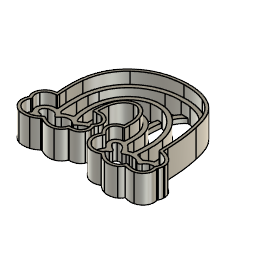
Rainbow v8 (Autodesk Fusion 360 design; units mm, degrees)
Autodesk Fusion 360 part; units mm, degrees
note: some values were not read from the file. Set by a fixed rule: which sketch regions a step uses.
(part 1 of 4)
sketch "Sketch1" plane through (0, 0, 0) normal (0, 0, 1) x (1, 0, 0)
  spline S0 degree 3 poles (40.6021, -45.3763) (39.7141, -45.1374) (38.685, -44.5376) (37.8366, -43.7642) knots 0 0 0 0 1 1 1 1
  line L0 (37.8366, -43.7642) -> (37.0528, -43.0498)
  line L1 (37.0528, -43.0498) -> (36.4497, -43.413)
  spline S1 degree 3 poles (36.4497, -43.413) (34.0687, -44.8468) (31.3596, -44.1594) (29.9199, -41.7563) knots 0 0 0 0 1 1 1 1
  spline S2 degree 3 poles (29.9199, -41.7563) (29.1248, -40.4292) (29.1935, -38.9614) (30.1335, -37.1915) knots 0 0 0 0 1 1 1 1
  line L2 (30.1335, -37.1915) -> (30.6349, -36.2474)
  line L3 (30.6349, -36.2474) -> (29.844, -35.4477)
  spline S3 degree 3 poles (29.844, -35.4477) (28.95, -34.5436) (28.6612, -33.9245) (28.6688, -32.9285) knots 0 0 0 0 1 1 1 1
  spline S4 degree 3 poles (28.6688, -32.9285) (28.6799, -31.4768) (29.8956, -30.2337) (31.6248, -29.9058) knots 0 0 0 0 1 1 1 1
  spline S5 degree 3 poles (31.6248, -29.9058) (31.9315, -29.8476) (32.2095, -29.7731) (32.2426, -29.7402) knots 0 0 0 0 1 1 1 1
  spline S6 degree 3 poles (32.2426, -29.7402) (32.2756, -29.7073) (32.3172, -28.7609) (32.3351, -27.6372) knots 0 0 0 0 1 1 1 1
  spline S7 degree 3 poles (32.3351, -27.6372) (32.3724, -25.2889) (32.226, -24.0781) (31.7223, -22.5668) knots 0 0 0 0 1 1 1 1
  spline S8 degree 3 poles (31.7223, -22.5668) (31.0329, -20.4985) (29.7724, -18.9275) (28.1619, -18.1295) knots 0 0 0 0 1 1 1 1
  spline S9 degree 3 poles (28.1619, -18.1295) (26.9869, -17.5472) (26.1291, -17.4128) (25.0253, -17.6379) knots 0 0 0 0 1 1 1 1
  spline S10 degree 3 poles (25.0253, -17.6379) (22.1239, -18.2295) (19.9977, -20.7694) (19.2274, -24.5637) knots 0 0 0 0 1 1 1 1
  spline S11 degree 3 poles (19.2274, -24.5637) (18.8969, -26.1921) (18.6739, -29.7666) (18.8842, -30.0674) knots 0 0 0 0 1 1 1 1
  spline S12 degree 3 poles (18.8842, -30.0674) (18.9324, -30.1364) (19.5594, -30.1752) (20.5764, -30.1721) knots 0 0 0 0 1 1 1 1
  spline S13 degree 3 poles (20.5764, -30.1721) (22.0397, -30.1678) (22.246, -30.1902) (22.7653, -30.4097) knots 0 0 0 0 1 1 1 1
  spline S14 degree 3 poles (22.7653, -30.4097) (24.0541, -30.9546) (24.7351, -31.7681) (24.8235, -32.8684) knots 0 0 0 0 1 1 1 1
  spline S15 degree 3 poles (24.8235, -32.8684) (24.8681, -33.424) (24.8348, -33.6203) (24.6146, -34.1013) knots 0 0 0 0 1 1 1 1
  spline S16 degree 3 poles (24.6146, -34.1013) (24.4706, -34.4159) (24.1763, -34.8686) (23.9606, -35.1073) knots 0 0 0 0 1 1 1 1
  line L4 (23.9606, -35.1073) -> (23.5686, -35.5413)
  line L5 (23.5686, -35.5413) -> (23.8705, -36.1371)
  spline S17 degree 3 poles (23.8705, -36.1371) (24.1088, -36.6075) (24.1803, -36.9044) (24.2098, -37.5469) knots 0 0 0 0 1 1 1 1
  spline S18 degree 3 poles (24.2098, -37.5469) (24.2439, -38.2891) (24.2182, -38.4195) (23.9188, -39.0278) knots 0 0 0 0 1 1 1 1
  spline S19 degree 3 poles (23.9188, -39.0278) (23.2828, -40.3197) (22.3235, -40.8384) (20.4042, -40.9282) knots 0 0 0 0 1 1 1 1
  line L6 (20.4042, -40.9282) -> (19.2417, -40.9826)
  line L7 (19.2417, -40.9826) -> (19.1816, -41.2833)
  spline S20 degree 3 poles (19.1816, -41.2833) (18.9486, -42.4484) (17.823, -43.6952) (16.6466, -44.0912) knots 0 0 0 0 1 1 1 1
  spline S21 degree 3 poles (16.6466, -44.0912) (15.1238, -44.6038) (13.5396, -44.3544) (11.5251, -43.2849) knots 0 0 0 0 1 1 1 1
  spline S22 degree 3 poles (11.5251, -43.2849) (10.3126, -42.6412) (10.4824, -42.625) (9.5048, -43.4776) knots 0 0 0 0 1 1 1 1
  spline S23 degree 3 poles (9.5048, -43.4776) (8.7123, -44.1689) (7.8391, -44.6696) (6.8696, -44.9888) knots 0 0 0 0 1 1 1 1
  spline S24 degree 3 poles (6.8696, -44.9888) (5.7759, -45.3488) (3.9668, -45.3933) (3.0651, -45.0822) knots 0 0 0 0 1 1 1 1
  spline S25 degree 3 poles (3.0651, -45.0822) (0.3591, -44.1486) (-0.7772, -41.3233) (0.6383, -39.0481) knots 0 0 0 0 1 1 1 1
  line L8 (0.6383, -39.0481) -> (0.884, -38.6532)
  line L9 (0.884, -38.6532) -> (0.5251, -38.0579)
  spline S26 degree 3 poles (0.5251, -38.0579) (-0.1869, -36.8769) (-0.2404, -35.9922) (0.3271, -34.7796) knots 0 0 0 0 1 1 1 1
  spline S27 degree 3 poles (0.3271, -34.7796) (1.1017, -33.1242) (2.7938, -32.1034) (4.7746, -32.0964) knots 0 0 0 0 1 1 1 1
  line L10 (4.7746, -32.0964) -> (5.2854, -32.0946)
  line L11 (5.2854, -32.0946) -> (5.222, -31.0262)
  spline S28 degree 3 poles (5.222, -31.0262) (5.1871, -30.4386) (5.1039, -29.1135) (5.0371, -28.0816) knots 0 0 0 0 1 1 1 1
  spline S29 degree 3 poles (5.0371, -28.0816) (4.8966, -25.9098) (4.9658, -22.8542) (5.1997, -20.8963) knots 0 0 0 0 1 1 1 1
  spline S30 degree 3 poles (5.1997, -20.8963) (5.8689, -15.2961) (8.1545, -10.5999) (11.9514, -7.0234) knots 0 0 0 0 1 1 1 1
  spline S31 degree 3 poles (11.9514, -7.0234) (16.4317, -2.8033) (22.1029, -0.554) (28.8108, -0.3366) knots 0 0 0 0 1 1 1 1
  spline S32 degree 3 poles (28.8108, -0.3366) (32.5622, -0.2151) (35.8702, -0.8038) (38.5701, -2.0736) knots 0 0 0 0 1 1 1 1
  spline S33 degree 3 poles (38.5701, -2.0736) (39.9873, -2.7401) (40.9328, -3.3672) (41.9013, -4.2831) knots 0 0 0 0 1 1 1 1
  spline S34 degree 3 poles (41.9013, -4.2831) (44.1778, -6.4358) (45.3916, -9.0372) (46.5245, -14.1912) knots 0 0 0 0 1 1 1 1
  spline S35 degree 3 poles (46.5245, -14.1912) (47.5435, -18.8273) (47.9159, -21.9078) (48.1971, -28.0295) knots 0 0 0 0 1 1 1 1
  spline S36 degree 3 poles (48.1971, -28.0295) (48.259, -29.3767) (48.3316, -30.5812) (48.3583, -30.7061) knots 0 0 0 0 1 1 1 1
  spline S37 degree 3 poles (48.3583, -30.7061) (48.3975, -30.889) (48.524, -30.9562) (49.0062, -31.0504) knots 0 0 0 0 1 1 1 1
  spline S38 degree 3 poles (49.0062, -31.0504) (51.4412, -31.526) (53.0985, -32.5346) (53.8053, -33.9708) knots 0 0 0 0 1 1 1 1
  spline S39 degree 3 poles (53.8053, -33.9708) (54.0458, -34.4594) (54.0871, -34.6749) (54.0852, -35.4301) knots 0 0 0 0 1 1 1 1
  spline S40 degree 3 poles (54.0852, -35.4301) (54.0832, -36.197) (54.0369, -36.4233) (53.7407, -37.1142) knots 0 0 0 0 1 1 1 1
  line L12 (53.7407, -37.1142) -> (53.3985, -37.9124)
  line L13 (53.3985, -37.9124) -> (53.5734, -38.5139)
  spline S41 degree 3 poles (53.5734, -38.5139) (54.1518, -40.5038) (52.8727, -42.5116) (50.6477, -43.1059) knots 0 0 0 0 1 1 1 1
  spline S42 degree 3 poles (50.6477, -43.1059) (49.6551, -43.3711) (48.4974, -43.2512) (46.8656, -42.7141) knots 0 0 0 0 1 1 1 1
  spline S43 degree 3 poles (46.8656, -42.7141) (46.1378, -42.4746) (45.9769, -42.523) (45.8572, -43.0173) knots 0 0 0 0 1 1 1 1
  spline S44 degree 3 poles (45.8572, -43.0173) (45.7413, -43.4966) (45.0944, -44.3751) (44.5754, -44.758) knots 0 0 0 0 1 1 1 1
  spline S45 degree 3 poles (44.5754, -44.758) (43.5936, -45.4825) (41.9487, -45.7385) (40.6021, -45.3763) knots 0 0 0 0 1 1 1 1
  spline S46 degree 3 poles (43.1464, -43.5675) (43.6121, -43.3637) (44.0986, -42.8484) (44.1975, -42.454) knots 0 0 0 0 1 1 1 1
  spline S47 degree 3 poles (44.1975, -42.454) (44.2329, -42.313) (44.2296, -41.9062) (44.1901, -41.55) knots 0 0 0 0 1 1 1 1
  spline S48 degree 3 poles (44.1901, -41.55) (44.0616, -40.3913) (44.0787, -40.2083) (44.3356, -40.0003) knots 0 0 0 0 1 1 1 1
  spline S49 degree 3 poles (44.3356, -40.0003) (44.7112, -39.6961) (45.1086, -39.7683) (46.0893, -40.3188) knots 0 0 0 0 1 1 1 1
  spline S50 degree 3 poles (46.0893, -40.3188) (47.5056, -41.1136) (48.2545, -41.3947) (49.1098, -41.4522) knots 0 0 0 0 1 1 1 1
  spline S51 degree 3 poles (49.1098, -41.4522) (50.0601, -41.5161) (50.6688, -41.3509) (51.2194, -40.8796) knots 0 0 0 0 1 1 1 1
  spline S52 degree 3 poles (51.2194, -40.8796) (51.7463, -40.4286) (51.9622, -40.0221) (51.9699, -39.4669) knots 0 0 0 0 1 1 1 1
  spline S53 degree 3 poles (51.9699, -39.4669) (51.9747, -39.1179) (51.9177, -38.9851) (51.6667, -38.7609) knots 0 0 0 0 1 1 1 1
  spline S54 degree 3 poles (51.6667, -38.7609) (51.4967, -38.6089) (51.1707, -38.4548) (50.9423, -38.4183) knots 0 0 0 0 1 1 1 1
  spline S55 degree 3 poles (50.9423, -38.4183) (50.0539, -38.2762) (49.4995, -37.6121) (49.7804, -37.0264) knots 0 0 0 0 1 1 1 1
  spline S56 degree 3 poles (49.7804, -37.0264) (49.9949, -36.579) (50.335, -36.453) (51.1465, -36.5202) knots 0 0 0 0 1 1 1 1
  spline S57 degree 3 poles (51.1465, -36.5202) (51.7992, -36.5743) (51.8736, -36.5589) (52.1107, -36.3219) knots 0 0 0 0 1 1 1 1
  spline S58 degree 3 poles (52.1107, -36.3219) (52.632, -35.8005) (52.3398, -34.5008) (51.5692, -33.913) knots 0 0 0 0 1 1 1 1
  spline S59 degree 3 poles (51.5692, -33.913) (50.1664, -32.8431) (48.1142, -32.4761) (46.4453, -32.9969) knots 0 0 0 0 1 1 1 1
  spline S60 degree 3 poles (46.4453, -32.9969) (45.8057, -33.1965) (44.9544, -33.904) (44.6602, -34.4802) knots 0 0 0 0 1 1 1 1
  spline S61 degree 3 poles (44.6602, -34.4802) (44.2129, -35.3568) (43.7112, -35.4679) (42.8564, -34.8799) knots 0 0 0 0 1 1 1 1
  spline S62 degree 3 poles (42.8564, -34.8799) (42.5554, -34.6729) (42.0276, -34.3719) (41.6837, -34.2111) knots 0 0 0 0 1 1 1 1
  spline S63 degree 3 poles (41.6837, -34.2111) (41.1075, -33.9417) (40.9598, -33.9187) (39.8075, -33.9187) knots 0 0 0 0 1 1 1 1
  line L14 (39.8075, -33.9187) -> (38.5567, -33.9187)
  line L15 (38.5567, -33.9187) -> (37.6186, -34.4148)
  spline S64 degree 3 poles (37.6186, -34.4148) (37.1026, -34.6877) (36.539, -34.9376) (36.3661, -34.9702) knots 0 0 0 0 1 1 1 1
  spline S65 degree 3 poles (36.3661, -34.9702) (35.922, -35.0539) (35.5337, -34.7143) (35.1462, -33.9031) knots 0 0 0 0 1 1 1 1
  spline S66 degree 3 poles (35.1462, -33.9031) (34.2767, -32.0829) (32.5077, -31.1785) (31.2082, -31.8899) knots 0 0 0 0 1 1 1 1
  spline S67 degree 3 poles (31.2082, -31.8899) (30.5745, -32.2368) (30.2974, -32.7818) (30.4669, -33.3475) knots 0 0 0 0 1 1 1 1
  spline S68 degree 3 poles (30.4669, -33.3475) (30.6161, -33.8457) (31.3598, -34.532) (32.2646, -35.0067) knots 0 0 0 0 1 1 1 1
  spline S69 degree 3 poles (32.2646, -35.0067) (33.1402, -35.466) (33.3971, -35.7096) (33.3971, -36.0805) knots 0 0 0 0 1 1 1 1
  spline S70 degree 3 poles (33.3971, -36.0805) (33.3971, -36.501) (33.238, -36.7542) (32.8468, -36.9565) knots 0 0 0 0 1 1 1 1
  spline S71 degree 3 poles (32.8468, -36.9565) (31.0444, -37.8883) (30.5759, -39.9699) (31.8443, -41.4109) knots 0 0 0 0 1 1 1 1
  spline S72 degree 3 poles (31.8443, -41.4109) (32.3815, -42.0212) (32.9483, -42.3169) (33.7139, -42.3863) knots 0 0 0 0 1 1 1 1
  spline S73 degree 3 poles (33.7139, -42.3863) (34.5937, -42.4661) (35.2523, -42.2098) (36.037, -41.4824) knots 0 0 0 0 1 1 1 1
  spline S74 degree 3 poles (36.037, -41.4824) (36.3909, -41.1543) (36.763, -40.8557) (36.8638, -40.8189) knots 0 0 0 0 1 1 1 1
  spline S75 degree 3 poles (36.8638, -40.8189) (37.192, -40.6989) (37.5089, -40.9167) (38.6147, -42.0227) knots 0 0 0 0 1 1 1 1
  spline S76 degree 3 poles (38.6147, -42.0227) (39.4081, -42.8162) (39.8679, -43.1882) (40.3105, -43.3948) knots 0 0 0 0 1 1 1 1
  spline S77 degree 3 poles (40.3105, -43.3948) (41.3954, -43.901) (42.2636, -43.9539) (43.1464, -43.5675) knots 0 0 0 0 1 1 1 1
  spline S78 degree 3 poles (6.3837, -43.2874) (7.3845, -42.9564) (8.1509, -42.4223) (9.1149, -41.384) knots 0 0 0 0 1 1 1 1
  spline S79 degree 3 poles (9.1149, -41.384) (9.6604, -40.7965) (9.9744, -40.5375) (10.1414, -40.5375) knots 0 0 0 0 1 1 1 1
  spline S80 degree 3 poles (10.1414, -40.5375) (10.2736, -40.5375) (10.8079, -40.801) (11.3285, -41.1231) knots 0 0 0 0 1 1 1 1
  spline S81 degree 3 poles (11.3285, -41.1231) (12.8148, -42.0424) (13.5925, -42.3956) (14.4099, -42.5224) knots 0 0 0 0 1 1 1 1
  spline S82 degree 3 poles (14.4099, -42.5224) (15.7434, -42.7294) (16.8719, -42.2963) (17.2889, -41.4175) knots 0 0 0 0 1 1 1 1
  spline S83 degree 3 poles (17.2889, -41.4175) (17.4425, -41.0937) (17.464, -40.8751) (17.4081, -40.2046) knots 0 0 0 0 1 1 1 1
  spline S84 degree 3 poles (17.4081, -40.2046) (17.3434, -39.4284) (17.3531, -39.3735) (17.5983, -39.1282) knots 0 0 0 0 1 1 1 1
  spline S85 degree 3 poles (17.5983, -39.1282) (17.8995, -38.827) (18.0838, -38.8152) (19.1861, -39.0261) knots 0 0 0 0 1 1 1 1
  spline S86 degree 3 poles (19.1861, -39.0261) (21.2987, -39.4304) (22.4511, -38.9297) (22.4522, -37.607) knots 0 0 0 0 1 1 1 1
  spline S87 degree 3 poles (22.4522, -37.607) (22.4529, -36.7454) (21.8377, -36.2639) (20.7361, -36.2639) knots 0 0 0 0 1 1 1 1
  spline S88 degree 3 poles (20.7361, -36.2639) (20.0382, -36.2639) (19.7425, -36.0347) (19.7425, -35.4937) knots 0 0 0 0 1 1 1 1
  spline S89 degree 3 poles (19.7425, -35.4937) (19.7425, -34.9001) (19.9962, -34.7075) (21.0588, -34.4943) knots 0 0 0 0 1 1 1 1
  spline S90 degree 3 poles (21.0588, -34.4943) (22.1331, -34.2788) (22.5478, -34.0955) (22.8603, -33.6982) knots 0 0 0 0 1 1 1 1
  spline S91 degree 3 poles (22.8603, -33.6982) (23.5958, -32.7632) (22.5543, -31.8861) (20.7083, -31.8861) knots 0 0 0 0 1 1 1 1
  spline S92 degree 3 poles (20.7083, -31.8861) (18.9346, -31.8861) (17.432, -32.5128) (15.9552, -33.8684) knots 0 0 0 0 1 1 1 1
  spline S93 degree 3 poles (15.9552, -33.8684) (15.4567, -34.326) (14.9608, -34.7004) (14.8533, -34.7004) knots 0 0 0 0 1 1 1 1
  spline S94 degree 3 poles (14.8533, -34.7004) (14.7458, -34.7004) (14.4299, -34.5351) (14.1513, -34.333) knots 0 0 0 0 1 1 1 1
  spline S95 degree 3 poles (14.1513, -34.333) (13.8727, -34.1309) (13.3868, -33.8381) (13.0715, -33.6822) knots 0 0 0 0 1 1 1 1
  spline S96 degree 3 poles (13.0715, -33.6822) (11.8711, -33.0889) (10.2509, -33.3985) (9.352, -34.393) knots 0 0 0 0 1 1 1 1
  spline S97 degree 3 poles (9.352, -34.393) (8.4004, -35.4459) (8.1864, -35.6385) (7.9683, -35.6385) knots 0 0 0 0 1 1 1 1
  spline S98 degree 3 poles (7.9683, -35.6385) (7.7171, -35.6385) (7.2977, -35.2383) (6.9738, -34.6891) knots 0 0 0 0 1 1 1 1
  spline S99 degree 3 poles (6.9738, -34.6891) (6.4989, -33.8843) (4.3788, -33.6094) (3.2207, -34.2025) knots 0 0 0 0 1 1 1 1
  spline S100 degree 3 poles (3.2207, -34.2025) (1.9483, -34.8542) (1.3752, -36.0623) (1.9202, -36.9441) knots 0 0 0 0 1 1 1 1
  spline S101 degree 3 poles (1.9202, -36.9441) (2.1572, -37.3277) (2.6853, -37.619) (3.1435, -37.619) knots 0 0 0 0 1 1 1 1
  spline S102 degree 3 poles (3.1435, -37.619) (3.8871, -37.619) (4.3159, -37.943) (4.3159, -38.505) knots 0 0 0 0 1 1 1 1
  spline S103 degree 3 poles (4.3159, -38.505) (4.3159, -39.0685) (4.1681, -39.1932) (3.1927, -39.4522) knots 0 0 0 0 1 1 1 1
  spline S104 degree 3 poles (3.1927, -39.4522) (2.8902, -39.5325) (2.529, -39.6727) (2.39, -39.7638) knots 0 0 0 0 1 1 1 1
  spline S105 degree 3 poles (2.39, -39.7638) (2.0795, -39.9672) (1.7097, -40.7046) (1.7111, -41.1177) knots 0 0 0 0 1 1 1 1
  spline S106 degree 3 poles (1.7111, -41.1177) (1.7137, -41.8847) (2.5286, -42.9734) (3.3605, -43.321) knots 0 0 0 0 1 1 1 1
  spline S107 degree 3 poles (3.3605, -43.321) (4.2972, -43.7123) (5.127, -43.7031) (6.3837, -43.2874) knots 0 0 0 0 1 1 1 1
  spline S108 degree 3 poles (8.705, -32.6248) (9.2851, -32.2374) (9.8665, -32.0076) (11.2214, -31.6303) knots 0 0 0 0 1 1 1 1
  spline S109 degree 3 poles (11.2214, -31.6303) (11.8742, -31.4485) (11.8914, -31.4155) (11.7143, -30.6874) knots 0 0 0 0 1 1 1 1
  spline S110 degree 3 poles (11.7143, -30.6874) (10.9845, -27.6875) (10.9096, -23.7891) (11.5242, -20.7853) knots 0 0 0 0 1 1 1 1
  spline S111 degree 3 poles (11.5242, -20.7853) (12.8947, -14.087) (17.7674, -9.0084) (23.8364, -7.9527) knots 0 0 0 0 1 1 1 1
  spline S112 degree 3 poles (23.8364, -7.9527) (24.5674, -7.8255) (25.2101, -7.7982) (26.5177, -7.8388) knots 0 0 0 0 1 1 1 1
  spline S113 degree 3 poles (26.5177, -7.8388) (28.4619, -7.8992) (29.3901, -8.1006) (31.078, -8.8283) knots 0 0 0 0 1 1 1 1
  spline S114 degree 3 poles (31.078, -8.8283) (35.3425, -10.6668) (38.7599, -15.2726) (39.9599, -20.7989) knots 0 0 0 0 1 1 1 1
  spline S115 degree 3 poles (39.9599, -20.7989) (40.381, -22.7381) (40.5138, -24.5489) (40.4444, -27.4041) knots 0 0 0 0 1 1 1 1
  spline S116 degree 3 poles (40.4444, -27.4041) (40.4089, -28.866) (40.3511, -30.4904) (40.316, -31.014) knots 0 0 0 0 1 1 1 1
  line L16 (40.316, -31.014) -> (40.2522, -31.966)
  line L17 (40.2522, -31.966) -> (41.7662, -32.4472)
  spline S117 degree 3 poles (41.7662, -32.4472) (42.5989, -32.7119) (43.3335, -32.9285) (43.3985, -32.9285) knots 0 0 0 0 1 1 1 1
  spline S118 degree 3 poles (43.3985, -32.9285) (43.4636, -32.9285) (43.808, -32.6862) (44.1638, -32.39) knots 0 0 0 0 1 1 1 1
  spline S119 degree 3 poles (44.1638, -32.39) (44.5196, -32.0939) (45.2044, -31.6627) (45.6856, -31.4317) knots 0 0 0 0 1 1 1 1
  line L18 (45.6856, -31.4317) -> (46.5605, -31.0119)
  line L19 (46.5605, -31.0119) -> (46.4885, -28.8171)
  spline S120 degree 3 poles (46.4885, -28.8171) (46.2828, -22.5508) (45.6972, -17.9425) (44.4939, -13.1206) knots 0 0 0 0 1 1 1 1
  spline S121 degree 3 poles (44.4939, -13.1206) (43.6086, -9.573) (42.6843, -7.6473) (41.0419, -5.9282) knots 0 0 0 0 1 1 1 1
  spline S122 degree 3 poles (41.0419, -5.9282) (39.2602, -4.0633) (36.9993, -2.991) (33.5472, -2.3735) knots 0 0 0 0 1 1 1 1
  spline S123 degree 3 poles (33.5472, -2.3735) (32.3588, -2.1609) (31.8638, -2.1321) (29.3841, -2.1308) knots 0 0 0 0 1 1 1 1
  spline S124 degree 3 poles (29.3841, -2.1308) (26.2893, -2.1292) (25.7344, -2.1938) (23.1155, -2.861) knots 0 0 0 0 1 1 1 1
  spline S125 degree 3 poles (23.1155, -2.861) (15.8271, -4.7179) (10.0738, -9.8891) (7.9282, -16.5117) knots 0 0 0 0 1 1 1 1
  spline S126 degree 3 poles (7.9282, -16.5117) (7.4178, -18.087) (7.2808, -18.6726) (7.0133, -20.4204) knots 0 0 0 0 1 1 1 1
  spline S127 degree 3 poles (7.0133, -20.4204) (6.814, -21.7234) (6.7809, -22.3775) (6.7737, -25.1631) knots 0 0 0 0 1 1 1 1
  spline S128 degree 3 poles (6.7737, -25.1631) (6.7643, -28.8189) (6.9545, -31.8997) (7.2227, -32.4341) knots 0 0 0 0 1 1 1 1
  spline S129 degree 3 poles (7.2227, -32.4341) (7.3731, -32.7338) (7.7563, -33.027) (8.0031, -33.0312) knots 0 0 0 0 1 1 1 1
  spline S130 degree 3 poles (8.0031, -33.0312) (8.0532, -33.032) (8.369, -32.8492) (8.705, -32.6248) knots 0 0 0 0 1 1 1 1
  spline S131 degree 3 poles (37.5865, -32.4424) (38.0054, -32.2897) (38.358, -32.1588) (38.3699, -32.1514) knots 0 0 0 0 1 1 1 1
  spline S132 degree 3 poles (38.3699, -32.1514) (38.3819, -32.1441) (38.4663, -31.4364) (38.5576, -30.5789) knots 0 0 0 0 1 1 1 1
  spline S133 degree 3 poles (38.5576, -30.5789) (38.7576, -28.7005) (38.787, -24.9492) (38.613, -23.4953) knots 0 0 0 0 1 1 1 1
  spline S134 degree 3 poles (38.613, -23.4953) (38.0797, -19.0373) (36.5859, -15.601) (34.0858, -13.0806) knots 0 0 0 0 1 1 1 1
  spline S135 degree 3 poles (34.0858, -13.0806) (32.465, -11.4468) (30.6163, -10.3222) (28.7127, -9.8123) knots 0 0 0 0 1 1 1 1
  spline S136 degree 3 poles (28.7127, -9.8123) (27.353, -9.4481) (25.087, -9.4274) (23.6217, -9.7658) knots 0 0 0 0 1 1 1 1
  spline S137 degree 3 poles (23.6217, -9.7658) (21.0994, -10.3485) (19.0072, -11.5487) (17.1769, -13.463) knots 0 0 0 0 1 1 1 1
  spline S138 degree 3 poles (17.1769, -13.463) (13.6018, -17.2023) (12.102, -22.8928) (13.1278, -28.8262) knots 0 0 0 0 1 1 1 1
  spline S139 degree 3 poles (13.1278, -28.8262) (13.3528, -30.1278) (13.671, -31.4351) (13.8593, -31.832) knots 0 0 0 0 1 1 1 1
  spline S140 degree 3 poles (13.8593, -31.832) (14.0085, -32.1465) (14.374, -32.4073) (14.6654, -32.4073) knots 0 0 0 0 1 1 1 1
  spline S141 degree 3 poles (14.6654, -32.4073) (14.734, -32.4073) (15.313, -32.0502) (15.9519, -31.6138) knots 0 0 0 0 1 1 1 1
  line L20 (15.9519, -31.6138) -> (17.1137, -30.8202)
  line L21 (17.1137, -30.8202) -> (17.1634, -28.2522)
  spline S142 degree 3 poles (17.1634, -28.2522) (17.2317, -24.7162) (17.5594, -23.0905) (18.6473, -20.8895) knots 0 0 0 0 1 1 1 1
  spline S143 degree 3 poles (18.6473, -20.8895) (19.9291, -18.2961) (21.9531, -16.557) (24.3463, -15.9928) knots 0 0 0 0 1 1 1 1
  spline S144 degree 3 poles (24.3463, -15.9928) (25.1987, -15.7919) (26.7215, -15.7913) (27.512, -15.9915) knots 0 0 0 0 1 1 1 1
  spline S145 degree 3 poles (27.512, -15.9915) (30.0811, -16.6424) (32.4074, -19.0232) (33.3899, -22.0071) knots 0 0 0 0 1 1 1 1
  spline S146 degree 3 poles (33.3899, -22.0071) (33.9317, -23.6526) (34.039, -24.4827) (34.0972, -27.4794) knots 0 0 0 0 1 1 1 1
  line L22 (34.0972, -27.4794) -> (34.1523, -30.317)
  line L23 (34.1523, -30.317) -> (34.6867, -30.7314)
  spline S147 degree 3 poles (34.6867, -30.7314) (34.9807, -30.9594) (35.5718, -31.5) (36.0003, -31.9329) knots 0 0 0 0 1 1 1 1
  spline S148 degree 3 poles (36.0003, -31.9329) (36.4288, -32.3658) (36.7897, -32.72) (36.8022, -32.72) knots 0 0 0 0 1 1 1 1
  spline S149 degree 3 poles (36.8022, -32.72) (36.8147, -32.72) (37.1676, -32.5951) (37.5865, -32.4424) knots 0 0 0 0 1 1 1 1
  spline S150 degree 3 poles (40.6021, -45.3763) (39.7141, -45.1374) (38.685, -44.5376) (37.8366, -43.7642) knots 0 0 0 0 1 1 1 1
  line L24 (37.8366, -43.7642) -> (37.0528, -43.0498)
  line L25 (37.0528, -43.0498) -> (36.4497, -43.413)
  spline S151 degree 3 poles (36.4497, -43.413) (34.0687, -44.8468) (31.3596, -44.1594) (29.9199, -41.7563) knots 0 0 0 0 1 1 1 1
  spline S152 degree 3 poles (29.9199, -41.7563) (29.1248, -40.4292) (29.1935, -38.9614) (30.1335, -37.1915) knots 0 0 0 0 1 1 1 1
  line L26 (30.1335, -37.1915) -> (30.6349, -36.2474)
  line L27 (30.6349, -36.2474) -> (29.844, -35.4477)
  spline S153 degree 3 poles (29.844, -35.4477) (28.95, -34.5436) (28.6612, -33.9245) (28.6688, -32.9285) knots 0 0 0 0 1 1 1 1
  spline S154 degree 3 poles (28.6688, -32.9285) (28.6799, -31.4768) (29.8956, -30.2337) (31.6248, -29.9058) knots 0 0 0 0 1 1 1 1
  spline S155 degree 3 poles (31.6248, -29.9058) (31.9315, -29.8476) (32.2095, -29.7731) (32.2426, -29.7402) knots 0 0 0 0 1 1 1 1
  spline S156 degree 3 poles (32.2426, -29.7402) (32.2756, -29.7073) (32.3172, -28.7609) (32.3351, -27.6372) knots 0 0 0 0 1 1 1 1
  spline S157 degree 3 poles (32.3351, -27.6372) (32.3724, -25.2889) (32.226, -24.0781) (31.7223, -22.5668) knots 0 0 0 0 1 1 1 1
  spline S158 degree 3 poles (31.7223, -22.5668) (31.0329, -20.4985) (29.7724, -18.9275) (28.1619, -18.1295) knots 0 0 0 0 1 1 1 1
  spline S159 degree 3 poles (28.1619, -18.1295) (26.9869, -17.5472) (26.1291, -17.4128) (25.0253, -17.6379) knots 0 0 0 0 1 1 1 1
  spline S160 degree 3 poles (25.0253, -17.6379) (22.1239, -18.2295) (19.9977, -20.7694) (19.2274, -24.5637) knots 0 0 0 0 1 1 1 1
  spline S161 degree 3 poles (19.2274, -24.5637) (18.8969, -26.1921) (18.6739, -29.7666) (18.8842, -30.0674) knots 0 0 0 0 1 1 1 1
  spline S162 degree 3 poles (18.8842, -30.0674) (18.9324, -30.1364) (19.5594, -30.1752) (20.5764, -30.1721) knots 0 0 0 0 1 1 1 1
  spline S163 degree 3 poles (20.5764, -30.1721) (22.0397, -30.1678) (22.246, -30.1902) (22.7653, -30.4097) knots 0 0 0 0 1 1 1 1
  spline S164 degree 3 poles (22.7653, -30.4097) (24.0541, -30.9546) (24.7351, -31.7681) (24.8235, -32.8684) knots 0 0 0 0 1 1 1 1
  spline S165 degree 3 poles (24.8235, -32.8684) (24.8681, -33.424) (24.8348, -33.6203) (24.6146, -34.1013) knots 0 0 0 0 1 1 1 1
  spline S166 degree 3 poles (24.6146, -34.1013) (24.4706, -34.4159) (24.1763, -34.8686) (23.9606, -35.1073) knots 0 0 0 0 1 1 1 1
  line L28 (23.9606, -35.1073) -> (23.5686, -35.5413)
  line L29 (23.5686, -35.5413) -> (23.8705, -36.1371)
  spline S167 degree 3 poles (23.8705, -36.1371) (24.1088, -36.6075) (24.1803, -36.9044) (24.2098, -37.5469) knots 0 0 0 0 1 1 1 1
  spline S168 degree 3 poles (24.2098, -37.5469) (24.2439, -38.2891) (24.2182, -38.4195) (23.9188, -39.0278) knots 0 0 0 0 1 1 1 1
  spline S169 degree 3 poles (23.9188, -39.0278) (23.2828, -40.3197) (22.3235, -40.8384) (20.4042, -40.9282) knots 0 0 0 0 1 1 1 1
  line L30 (20.4042, -40.9282) -> (19.2417, -40.9826)
  line L31 (19.2417, -40.9826) -> (19.1816, -41.2833)
  spline S170 degree 3 poles (19.1816, -41.2833) (18.9486, -42.4484) (17.823, -43.6952) (16.6466, -44.0912) knots 0 0 0 0 1 1 1 1
  spline S171 degree 3 poles (16.6466, -44.0912) (15.1238, -44.6038) (13.5396, -44.3544) (11.5251, -43.2849) knots 0 0 0 0 1 1 1 1
  spline S172 degree 3 poles (11.5251, -43.2849) (10.3126, -42.6412) (10.4824, -42.625) (9.5048, -43.4776) knots 0 0 0 0 1 1 1 1
  spline S173 degree 3 poles (9.5048, -43.4776) (8.7123, -44.1689) (7.8391, -44.6696) (6.8696, -44.9888) knots 0 0 0 0 1 1 1 1
  spline S174 degree 3 poles (6.8696, -44.9888) (5.7759, -45.3488) (3.9668, -45.3933) (3.0651, -45.0822) knots 0 0 0 0 1 1 1 1
  spline S175 degree 3 poles (3.0651, -45.0822) (0.3591, -44.1486) (-0.7772, -41.3233) (0.6383, -39.0481) knots 0 0 0 0 1 1 1 1
  line L32 (0.6383, -39.0481) -> (0.884, -38.6532)
  line L33 (0.884, -38.6532) -> (0.5251, -38.0579)
  spline S176 degree 3 poles (0.5251, -38.0579) (-0.1869, -36.8769) (-0.2404, -35.9922) (0.3271, -34.7796) knots 0 0 0 0 1 1 1 1
  spline S177 degree 3 poles (0.3271, -34.7796) (1.1017, -33.1242) (2.7938, -32.1034) (4.7746, -32.0964) knots 0 0 0 0 1 1 1 1
  line L34 (4.7746, -32.0964) -> (5.2854, -32.0946)
  line L35 (5.2854, -32.0946) -> (5.222, -31.0262)
  spline S178 degree 3 poles (5.222, -31.0262) (5.1871, -30.4386) (5.1039, -29.1135) (5.0371, -28.0816) knots 0 0 0 0 1 1 1 1
  spline S179 degree 3 poles (5.0371, -28.0816) (4.8966, -25.9098) (4.9658, -22.8542) (5.1997, -20.8963) knots 0 0 0 0 1 1 1 1
  spline S180 degree 3 poles (5.1997, -20.8963) (5.8689, -15.2961) (8.1545, -10.5999) (11.9514, -7.0234) knots 0 0 0 0 1 1 1 1
  spline S181 degree 3 poles (11.9514, -7.0234) (16.4317, -2.8033) (22.1029, -0.554) (28.8108, -0.3366) knots 0 0 0 0 1 1 1 1
  spline S182 degree 3 poles (28.8108, -0.3366) (32.5622, -0.2151) (35.8702, -0.8038) (38.5701, -2.0736) knots 0 0 0 0 1 1 1 1
  spline S183 degree 3 poles (38.5701, -2.0736) (39.9873, -2.7401) (40.9328, -3.3672) (41.9013, -4.2831) knots 0 0 0 0 1 1 1 1
  spline S184 degree 3 poles (41.9013, -4.2831) (44.1778, -6.4358) (45.3916, -9.0372) (46.5245, -14.1912) knots 0 0 0 0 1 1 1 1
  spline S185 degree 3 poles (46.5245, -14.1912) (47.5435, -18.8273) (47.9159, -21.9078) (48.1971, -28.0295) knots 0 0 0 0 1 1 1 1
  spline S186 degree 3 poles (48.1971, -28.0295) (48.259, -29.3767) (48.3316, -30.5812) (48.3583, -30.7061) knots 0 0 0 0 1 1 1 1
  spline S187 degree 3 poles (48.3583, -30.7061) (48.3975, -30.889) (48.524, -30.9562) (49.0062, -31.0504) knots 0 0 0 0 1 1 1 1
  spline S188 degree 3 poles (49.0062, -31.0504) (51.4412, -31.526) (53.0985, -32.5346) (53.8053, -33.9708) knots 0 0 0 0 1 1 1 1
  spline S189 degree 3 poles (53.8053, -33.9708) (54.0458, -34.4594) (54.0871, -34.6749) (54.0852, -35.4301) knots 0 0 0 0 1 1 1 1
  spline S190 degree 3 poles (54.0852, -35.4301) (54.0832, -36.197) (54.0369, -36.4233) (53.7407, -37.1142) knots 0 0 0 0 1 1 1 1
  line L36 (53.7407, -37.1142) -> (53.3985, -37.9124)
  line L37 (53.3985, -37.9124) -> (53.5734, -38.5139)
  spline S191 degree 3 poles (53.5734, -38.5139) (54.1518, -40.5038) (52.8727, -42.5116) (50.6477, -43.1059) knots 0 0 0 0 1 1 1 1
  spline S192 degree 3 poles (50.6477, -43.1059) (49.6551, -43.3711) (48.4974, -43.2512) (46.8656, -42.7141) knots 0 0 0 0 1 1 1 1
  spline S193 degree 3 poles (46.8656, -42.7141) (46.1378, -42.4746) (45.9769, -42.523) (45.8572, -43.0173) knots 0 0 0 0 1 1 1 1
  spline S194 degree 3 poles (45.8572, -43.0173) (45.7413, -43.4966) (45.0944, -44.3751) (44.5754, -44.758) knots 0 0 0 0 1 1 1 1
  spline S195 degree 3 poles (44.5754, -44.758) (43.5936, -45.4825) (41.9487, -45.7385) (40.6021, -45.3763) knots 0 0 0 0 1 1 1 1
  spline S196 degree 3 poles (43.1464, -43.5675) (43.6121, -43.3637) (44.0986, -42.8484) (44.1975, -42.454) knots 0 0 0 0 1 1 1 1
  spline S197 degree 3 poles (44.1975, -42.454) (44.2329, -42.313) (44.2296, -41.9062) (44.1901, -41.55) knots 0 0 0 0 1 1 1 1
  spline S198 degree 3 poles (44.1901, -41.55) (44.0616, -40.3913) (44.0787, -40.2083) (44.3356, -40.0003) knots 0 0 0 0 1 1 1 1
  spline S199 degree 3 poles (44.3356, -40.0003) (44.7112, -39.6961) (45.1086, -39.7683) (46.0893, -40.3188) knots 0 0 0 0 1 1 1 1
  spline S200 degree 3 poles (46.0893, -40.3188) (47.5056, -41.1136) (48.2545, -41.3947) (49.1098, -41.4522) knots 0 0 0 0 1 1 1 1
  spline S201 degree 3 poles (49.1098, -41.4522) (50.0601, -41.5161) (50.6688, -41.3509) (51.2194, -40.8796) knots 0 0 0 0 1 1 1 1
  spline S202 degree 3 poles (51.2194, -40.8796) (51.7463, -40.4286) (51.9622, -40.0221) (51.9699, -39.4669) knots 0 0 0 0 1 1 1 1
  spline S203 degree 3 poles (51.9699, -39.4669) (51.9747, -39.1179) (51.9177, -38.9851) (51.6667, -38.7609) knots 0 0 0 0 1 1 1 1
  spline S204 degree 3 poles (51.6667, -38.7609) (51.4967, -38.6089) (51.1707, -38.4548) (50.9423, -38.4183) knots 0 0 0 0 1 1 1 1
  spline S205 degree 3 poles (50.9423, -38.4183) (50.0539, -38.2762) (49.4995, -37.6121) (49.7804, -37.0264) knots 0 0 0 0 1 1 1 1
  spline S206 degree 3 poles (49.7804, -37.0264) (49.9949, -36.579) (50.335, -36.453) (51.1465, -36.5202) knots 0 0 0 0 1 1 1 1
  spline S207 degree 3 poles (51.1465, -36.5202) (51.7992, -36.5743) (51.8736, -36.5589) (52.1107, -36.3219) knots 0 0 0 0 1 1 1 1
  spline S208 degree 3 poles (52.1107, -36.3219) (52.632, -35.8005) (52.3398, -34.5008) (51.5692, -33.913) knots 0 0 0 0 1 1 1 1
  spline S209 degree 3 poles (51.5692, -33.913) (50.1664, -32.8431) (48.1142, -32.4761) (46.4453, -32.9969) knots 0 0 0 0 1 1 1 1
  spline S210 degree 3 poles (46.4453, -32.9969) (45.8057, -33.1965) (44.9544, -33.904) (44.6602, -34.4802) knots 0 0 0 0 1 1 1 1
  spline S211 degree 3 poles (44.6602, -34.4802) (44.2129, -35.3568) (43.7112, -35.4679) (42.8564, -34.8799) knots 0 0 0 0 1 1 1 1
  spline S212 degree 3 poles (42.8564, -34.8799) (42.5554, -34.6729) (42.0276, -34.3719) (41.6837, -34.2111) knots 0 0 0 0 1 1 1 1
  spline S213 degree 3 poles (41.6837, -34.2111) (41.1075, -33.9417) (40.9598, -33.9187) (39.8075, -33.9187) knots 0 0 0 0 1 1 1 1
  line L38 (39.8075, -33.9187) -> (38.5567, -33.9187)
  line L39 (38.5567, -33.9187) -> (37.6186, -34.4148)
  spline S214 degree 3 poles (37.6186, -34.4148) (37.1026, -34.6877) (36.539, -34.9376) (36.3661, -34.9702) knots 0 0 0 0 1 1 1 1
  spline S215 degree 3 poles (36.3661, -34.9702) (35.922, -35.0539) (35.5337, -34.7143) (35.1462, -33.9031) knots 0 0 0 0 1 1 1 1
  spline S216 degree 3 poles (35.1462, -33.9031) (34.2767, -32.0829) (32.5077, -31.1785) (31.2082, -31.8899) knots 0 0 0 0 1 1 1 1
  spline S217 degree 3 poles (31.2082, -31.8899) (30.5745, -32.2368) (30.2974, -32.7818) (30.4669, -33.3475) knots 0 0 0 0 1 1 1 1
  spline S218 degree 3 poles (30.4669, -33.3475) (30.6161, -33.8457) (31.3598, -34.532) (32.2646, -35.0067) knots 0 0 0 0 1 1 1 1
  spline S219 degree 3 poles (32.2646, -35.0067) (33.1402, -35.466) (33.3971, -35.7096) (33.3971, -36.0805) knots 0 0 0 0 1 1 1 1
  spline S220 degree 3 poles (33.3971, -36.0805) (33.3971, -36.501) (33.238, -36.7542) (32.8468, -36.9565) knots 0 0 0 0 1 1 1 1
  spline S221 degree 3 poles (32.8468, -36.9565) (31.0444, -37.8883) (30.5759, -39.9699) (31.8443, -41.4109) knots 0 0 0 0 1 1 1 1
  spline S222 degree 3 poles (31.8443, -41.4109) (32.3815, -42.0212) (32.9483, -42.3169) (33.7139, -42.3863) knots 0 0 0 0 1 1 1 1
  spline S223 degree 3 poles (33.7139, -42.3863) (34.5937, -42.4661) (35.2523, -42.2098) (36.037, -41.4824) knots 0 0 0 0 1 1 1 1
  spline S224 degree 3 poles (36.037, -41.4824) (36.3909, -41.1543) (36.763, -40.8557) (36.8638, -40.8189) knots 0 0 0 0 1 1 1 1
  spline S225 degree 3 poles (36.8638, -40.8189) (37.192, -40.6989) (37.5089, -40.9167) (38.6147, -42.0227) knots 0 0 0 0 1 1 1 1
  spline S226 degree 3 poles (38.6147, -42.0227) (39.4081, -42.8162) (39.8679, -43.1882) (40.3105, -43.3948) knots 0 0 0 0 1 1 1 1
  spline S227 degree 3 poles (40.3105, -43.3948) (41.3954, -43.901) (42.2636, -43.9539) (43.1464, -43.5675) knots 0 0 0 0 1 1 1 1
  spline S228 degree 3 poles (6.3837, -43.2874) (7.3845, -42.9564) (8.1509, -42.4223) (9.1149, -41.384) knots 0 0 0 0 1 1 1 1
  spline S229 degree 3 poles (9.1149, -41.384) (9.6604, -40.7965) (9.9744, -40.5375) (10.1414, -40.5375) knots 0 0 0 0 1 1 1 1
  spline S230 degree 3 poles (10.1414, -40.5375) (10.2736, -40.5375) (10.8079, -40.801) (11.3285, -41.1231) knots 0 0 0 0 1 1 1 1
  spline S231 degree 3 poles (11.3285, -41.1231) (12.8148, -42.0424) (13.5925, -42.3956) (14.4099, -42.5224) knots 0 0 0 0 1 1 1 1
  spline S232 degree 3 poles (14.4099, -42.5224) (15.7434, -42.7294) (16.8719, -42.2963) (17.2889, -41.4175) knots 0 0 0 0 1 1 1 1
  spline S233 degree 3 poles (17.2889, -41.4175) (17.4425, -41.0937) (17.464, -40.8751) (17.4081, -40.2046) knots 0 0 0 0 1 1 1 1
  spline S234 degree 3 poles (17.4081, -40.2046) (17.3434, -39.4284) (17.3531, -39.3735) (17.5983, -39.1282) knots 0 0 0 0 1 1 1 1
  spline S235 degree 3 poles (17.5983, -39.1282) (17.8995, -38.827) (18.0838, -38.8152) (19.1861, -39.0261) knots 0 0 0 0 1 1 1 1
  spline S236 degree 3 poles (19.1861, -39.0261) (21.2987, -39.4304) (22.4511, -38.9297) (22.4522, -37.607) knots 0 0 0 0 1 1 1 1
  spline S237 degree 3 poles (22.4522, -37.607) (22.4529, -36.7454) (21.8377, -36.2639) (20.7361, -36.2639) knots 0 0 0 0 1 1 1 1
  spline S238 degree 3 poles (20.7361, -36.2639) (20.0382, -36.2639) (19.7425, -36.0347) (19.7425, -35.4937) knots 0 0 0 0 1 1 1 1
  spline S239 degree 3 poles (19.7425, -35.4937) (19.7425, -34.9001) (19.9962, -34.7075) (21.0588, -34.4943) knots 0 0 0 0 1 1 1 1
  spline S240 degree 3 poles (21.0588, -34.4943) (22.1331, -34.2788) (22.5478, -34.0955) (22.8603, -33.6982) knots 0 0 0 0 1 1 1 1
  spline S241 degree 3 poles (22.8603, -33.6982) (23.5958, -32.7632) (22.5543, -31.8861) (20.7083, -31.8861) knots 0 0 0 0 1 1 1 1
  spline S242 degree 3 poles (20.7083, -31.8861) (18.9346, -31.8861) (17.432, -32.5128) (15.9552, -33.8684) knots 0 0 0 0 1 1 1 1
  spline S243 degree 3 poles (15.9552, -33.8684) (15.4567, -34.326) (14.9608, -34.7004) (14.8533, -34.7004) knots 0 0 0 0 1 1 1 1
  spline S244 degree 3 poles (14.8533, -34.7004) (14.7458, -34.7004) (14.4299, -34.5351) (14.1513, -34.333) knots 0 0 0 0 1 1 1 1
  spline S245 degree 3 poles (14.1513, -34.333) (13.8727, -34.1309) (13.3868, -33.8381) (13.0715, -33.6822) knots 0 0 0 0 1 1 1 1
  spline S246 degree 3 poles (13.0715, -33.6822) (11.8711, -33.0889) (10.2509, -33.3985) (9.352, -34.393) knots 0 0 0 0 1 1 1 1
  spline S247 degree 3 poles (9.352, -34.393) (8.4004, -35.4459) (8.1864, -35.6385) (7.9683, -35.6385) knots 0 0 0 0 1 1 1 1
  spline S248 degree 3 poles (7.9683, -35.6385) (7.7171, -35.6385) (7.2977, -35.2383) (6.9738, -34.6891) knots 0 0 0 0 1 1 1 1
  spline S249 degree 3 poles (6.9738, -34.6891) (6.4989, -33.8843) (4.3788, -33.6094) (3.2207, -34.2025) knots 0 0 0 0 1 1 1 1
  spline S250 degree 3 poles (3.2207, -34.2025) (1.9483, -34.8542) (1.3752, -36.0623) (1.9202, -36.9441) knots 0 0 0 0 1 1 1 1
  spline S251 degree 3 poles (1.9202, -36.9441) (2.1572, -37.3277) (2.6853, -37.619) (3.1435, -37.619) knots 0 0 0 0 1 1 1 1
  spline S252 degree 3 poles (3.1435, -37.619) (3.8871, -37.619) (4.3159, -37.943) (4.3159, -38.505) knots 0 0 0 0 1 1 1 1
  spline S253 degree 3 poles (4.3159, -38.505) (4.3159, -39.0685) (4.1681, -39.1932) (3.1927, -39.4522) knots 0 0 0 0 1 1 1 1
  spline S254 degree 3 poles (3.1927, -39.4522) (2.8902, -39.5325) (2.529, -39.6727) (2.39, -39.7638) knots 0 0 0 0 1 1 1 1
  spline S255 degree 3 poles (2.39, -39.7638) (2.0795, -39.9672) (1.7097, -40.7046) (1.7111, -41.1177) knots 0 0 0 0 1 1 1 1
  spline S256 degree 3 poles (1.7111, -41.1177) (1.7137, -41.8847) (2.5286, -42.9734) (3.3605, -43.321) knots 0 0 0 0 1 1 1 1
  spline S257 degree 3 poles (3.3605, -43.321) (4.2972, -43.7123) (5.127, -43.7031) (6.3837, -43.2874) knots 0 0 0 0 1 1 1 1
  spline S258 degree 3 poles (8.705, -32.6248) (9.2851, -32.2374) (9.8665, -32.0076) (11.2214, -31.6303) knots 0 0 0 0 1 1 1 1
  spline S259 degree 3 poles (11.2214, -31.6303) (11.8742, -31.4485) (11.8914, -31.4155) (11.7143, -30.6874) knots 0 0 0 0 1 1 1 1
  spline S260 degree 3 poles (11.7143, -30.6874) (10.9845, -27.6875) (10.9096, -23.7891) (11.5242, -20.7853) knots 0 0 0 0 1 1 1 1
  spline S261 degree 3 poles (11.5242, -20.7853) (12.8947, -14.087) (17.7674, -9.0084) (23.8364, -7.9527) knots 0 0 0 0 1 1 1 1
  spline S262 degree 3 poles (23.8364, -7.9527) (24.5674, -7.8255) (25.2101, -7.7982) (26.5177, -7.8388) knots 0 0 0 0 1 1 1 1
  spline S263 degree 3 poles (26.5177, -7.8388) (28.4619, -7.8992) (29.3901, -8.1006) (31.078, -8.8283) knots 0 0 0 0 1 1 1 1
  spline S264 degree 3 poles (31.078, -8.8283) (35.3425, -10.6668) (38.7599, -15.2726) (39.9599, -20.7989) knots 0 0 0 0 1 1 1 1
  spline S265 degree 3 poles (39.9599, -20.7989) (40.381, -22.7381) (40.5138, -24.5489) (40.4444, -27.4041) knots 0 0 0 0 1 1 1 1
  spline S266 degree 3 poles (40.4444, -27.4041) (40.4089, -28.866) (40.3511, -30.4904) (40.316, -31.014) knots 0 0 0 0 1 1 1 1
  line L40 (40.316, -31.014) -> (40.2522, -31.966)
  line L41 (40.2522, -31.966) -> (41.7662, -32.4472)
  spline S267 degree 3 poles (41.7662, -32.4472) (42.5989, -32.7119) (43.3335, -32.9285) (43.3985, -32.9285) knots 0 0 0 0 1 1 1 1
  spline S268 degree 3 poles (43.3985, -32.9285) (43.4636, -32.9285) (43.808, -32.6862) (44.1638, -32.39) knots 0 0 0 0 1 1 1 1
  spline S269 degree 3 poles (44.1638, -32.39) (44.5196, -32.0939) (45.2044, -31.6627) (45.6856, -31.4317) knots 0 0 0 0 1 1 1 1
  line L42 (45.6856, -31.4317) -> (46.5605, -31.0119)
  line L43 (46.5605, -31.0119) -> (46.4885, -28.8171)
  spline S270 degree 3 poles (46.4885, -28.8171) (46.2828, -22.5508) (45.6972, -17.9425) (44.4939, -13.1206) knots 0 0 0 0 1 1 1 1
  spline S271 degree 3 poles (44.4939, -13.1206) (43.6086, -9.573) (42.6843, -7.6473) (41.0419, -5.9282) knots 0 0 0 0 1 1 1 1
  spline S272 degree 3 poles (41.0419, -5.9282) (39.2602, -4.0633) (36.9993, -2.991) (33.5472, -2.3735) knots 0 0 0 0 1 1 1 1
  spline S273 degree 3 poles (33.5472, -2.3735) (32.3588, -2.1609) (31.8638, -2.1321) (29.3841, -2.1308) knots 0 0 0 0 1 1 1 1
  spline S274 degree 3 poles (29.3841, -2.1308) (26.2893, -2.1292) (25.7344, -2.1938) (23.1155, -2.861) knots 0 0 0 0 1 1 1 1
  spline S275 degree 3 poles (23.1155, -2.861) (15.8271, -4.7179) (10.0738, -9.8891) (7.9282, -16.5117) knots 0 0 0 0 1 1 1 1
  spline S276 degree 3 poles (7.9282, -16.5117) (7.4178, -18.087) (7.2808, -18.6726) (7.0133, -20.4204) knots 0 0 0 0 1 1 1 1
  spline S277 degree 3 poles (7.0133, -20.4204) (6.814, -21.7234) (6.7809, -22.3775) (6.7737, -25.1631) knots 0 0 0 0 1 1 1 1
  spline S278 degree 3 poles (6.7737, -25.1631) (6.7643, -28.8189) (6.9545, -31.8997) (7.2227, -32.4341) knots 0 0 0 0 1 1 1 1
  spline S279 degree 3 poles (7.2227, -32.4341) (7.3731, -32.7338) (7.7563, -33.027) (8.0031, -33.0312) knots 0 0 0 0 1 1 1 1
  spline S280 degree 3 poles (8.0031, -33.0312) (8.0532, -33.032) (8.369, -32.8492) (8.705, -32.6248) knots 0 0 0 0 1 1 1 1
  spline S281 degree 3 poles (37.5865, -32.4424) (38.0054, -32.2897) (38.358, -32.1588) (38.3699, -32.1514) knots 0 0 0 0 1 1 1 1
  spline S282 degree 3 poles (38.3699, -32.1514) (38.3819, -32.1441) (38.4663, -31.4364) (38.5576, -30.5789) knots 0 0 0 0 1 1 1 1
  spline S283 degree 3 poles (38.5576, -30.5789) (38.7576, -28.7005) (38.787, -24.9492) (38.613, -23.4953) knots 0 0 0 0 1 1 1 1
  spline S284 degree 3 poles (38.613, -23.4953) (38.0797, -19.0373) (36.5859, -15.601) (34.0858, -13.0806) knots 0 0 0 0 1 1 1 1
  spline S285 degree 3 poles (34.0858, -13.0806) (32.465, -11.4468) (30.6163, -10.3222) (28.7127, -9.8123) knots 0 0 0 0 1 1 1 1
  spline S286 degree 3 poles (28.7127, -9.8123) (27.353, -9.4481) (25.087, -9.4274) (23.6217, -9.7658) knots 0 0 0 0 1 1 1 1
  spline S287 degree 3 poles (23.6217, -9.7658) (21.0994, -10.3485) (19.0072, -11.5487) (17.1769, -13.463) knots 0 0 0 0 1 1 1 1
  spline S288 degree 3 poles (17.1769, -13.463) (13.6018, -17.2023) (12.102, -22.8928) (13.1278, -28.8262) knots 0 0 0 0 1 1 1 1
  spline S289 degree 3 poles (13.1278, -28.8262) (13.3528, -30.1278) (13.671, -31.4351) (13.8593, -31.832) knots 0 0 0 0 1 1 1 1
  spline S290 degree 3 poles (13.8593, -31.832) (14.0085, -32.1465) (14.374, -32.4073) (14.6654, -32.4073) knots 0 0 0 0 1 1 1 1
  spline S291 degree 3 poles (14.6654, -32.4073) (14.734, -32.4073) (15.313, -32.0502) (15.9519, -31.6138) knots 0 0 0 0 1 1 1 1
  line L44 (15.9519, -31.6138) -> (17.1137, -30.8202)
  line L45 (17.1137, -30.8202) -> (17.1634, -28.2522)
  spline S292 degree 3 poles (17.1634, -28.2522) (17.2317, -24.7162) (17.5594, -23.0905) (18.6473, -20.8895) knots 0 0 0 0 1 1 1 1
  spline S293 degree 3 poles (18.6473, -20.8895) (19.9291, -18.2961) (21.9531, -16.557) (24.3463, -15.9928) knots 0 0 0 0 1 1 1 1
  spline S294 degree 3 poles (24.3463, -15.9928) (25.1987, -15.7919) (26.7215, -15.7913) (27.512, -15.9915) knots 0 0 0 0 1 1 1 1
  spline S295 degree 3 poles (27.512, -15.9915) (30.0811, -16.6424) (32.4074, -19.0232) (33.3899, -22.0071) knots 0 0 0 0 1 1 1 1
  spline S296 degree 3 poles (33.3899, -22.0071) (33.9317, -23.6526) (34.039, -24.4827) (34.0972, -27.4794) knots 0 0 0 0 1 1 1 1
  line L46 (34.0972, -27.4794) -> (34.1523, -30.317)
  line L47 (34.1523, -30.317) -> (34.6867, -30.7314)
  spline S297 degree 3 poles (34.6867, -30.7314) (34.9807, -30.9594) (35.5718, -31.5) (36.0003, -31.9329) knots 0 0 0 0 1 1 1 1
  spline S298 degree 3 poles (36.0003, -31.9329) (36.4288, -32.3658) (36.7897, -32.72) (36.8022, -32.72) knots 0 0 0 0 1 1 1 1
  spline S299 degree 3 poles (36.8022, -32.72) (36.8147, -32.72) (37.1676, -32.5951) (37.5865, -32.4424) knots 0 0 0 0 1 1 1 1
  line L48 (54.6708, -37.9902) -> (54.6709, -37.9899)
  line L49 (55.2846, -35.2136) -> (55.2832, -35.6451)
  spline S300 degree 3 poles (11.1287, -6.1499) (15.8219, -1.7292) (21.8181, 0.6374) (28.7719, 0.8627) knots 0 0 0 0 1 1 1 1
  spline S301 degree 3 poles (28.7719, 0.8627) (32.6715, 0.9891) (36.1686, 0.3819) (39.0808, -0.9877) knots 0 0 0 0 1 1 1 1
  spline S302 degree 3 poles (39.0808, -0.9877) (40.5743, -1.6901) (41.6727, -2.4153) (42.7258, -3.4112) knots 0 0 0 0 1 1 1 1
  spline S303 degree 3 poles (42.7258, -3.4112) (44.4016, -4.9959) (45.589, -6.8874) (46.5056, -9.5421) (46.9414, -10.8042) (47.3249, -12.2429) (47.6965, -13.9335) knots 0 0 0 0 0.677783 0.677783 0.677783 1 1 1 1
  spline S304 degree 3 poles (47.6965, -13.9335) (48.7263, -18.6186) (49.1132, -21.8227) (49.3958, -27.9744) knots 0 0 0 0 1 1 1 1
  spline S305 degree 3 poles (49.3958, -27.9744) (49.4246, -28.6004) (49.4557, -29.1959) (49.4832, -29.6611) (49.4887, -29.7552) (49.4941, -29.8438) (49.4993, -29.9265) knots 0 0 0 0 0.46819 0.46819 0.46819 0.562944 0.562944 0.562944 0.562944
  spline S306 degree 3 poles (49.4993, -29.9265) (51.3935, -30.3328) (52.9435, -31.0564) (54.0116, -32.193) (54.363, -32.5669) (54.6579, -32.9856) (54.882, -33.4409) knots 0.033409 0.033409 0.033409 0.033409 0.760746 0.760746 0.760746 0.999997 0.999997 0.999997 0.999997
  spline S307 degree 3 poles (54.882, -33.4409) (55.0347, -33.7513) (55.1727, -34.0995) (55.2323, -34.4752) (55.2812, -34.7838) (55.2861, -35.0726) (55.2852, -35.4331) knots 0 0 0 0 0.549059 0.549059 0.549059 1 1 1 1
  spline S308 degree 3 poles (55.2852, -35.4332) (55.284, -35.8757) (55.2691, -36.2453) (55.1786, -36.6345) (55.1024, -36.9617) (54.9878, -37.2507) (54.8436, -37.5871) knots 0 0 0 0 0.543269 0.543269 0.543269 1 1 1 1
  line L50 (54.8436, -37.5871) -> (54.6708, -37.9902)
  line L51 (54.6708, -37.9902) -> (54.7256, -38.1789)
  spline S309 degree 3 poles (54.7256, -38.1789) (55.1949, -39.793) (54.7298, -41.4712) (53.6604, -42.6498) (52.9721, -43.4084) (52.0402, -43.976) (50.9574, -44.2653) knots 0 0 0 0 0.608426 0.608426 0.608426 1 1 1 1
  spline S310 degree 3 poles (50.9574, -44.2653) (49.8818, -44.5526) (48.7117, -44.4734) (47.3744, -44.1183) (47.178, -44.0661) (46.9771, -44.0079) (46.771, -43.9438) knots 0 0 0 0 0.824545 0.824545 0.824545 0.945665 0.945665 0.945665 0.945665
  spline S311 degree 3 poles (46.771, -43.9438) (46.7093, -44.062) (46.6405, -44.1796) (46.5676, -44.2944) (46.2623, -44.7749) (45.8902, -45.2321) (45.4363, -45.6075) (45.3884, -45.647) (45.3392, -45.6858) (45.2879, -45.7236) knots 0.223295 0.223295 0.223295 0.223295 0.361232 0.361232 0.361232 0.939053 0.939053 0.939053 1 1 1 1
  spline S312 degree 3 poles (45.2879, -45.7236) (44.2745, -46.4714) (42.9911, -46.772) (41.707, -46.737) (41.2318, -46.724) (40.7551, -46.6601) (40.2904, -46.5351) knots 0.000002 0.000002 0.000002 0.000002 0.729882 0.729882 0.729882 1 1 1 1
  spline S313 degree 3 poles (40.2904, -46.5351) (39.1403, -46.2258) (38.0053, -45.5417) (37.0282, -44.651) knots 0.000001 0.000001 0.000001 0.000001 1 1 1 1
  line L52 (37.0282, -44.651) -> (36.9035, -44.5374)
  spline S314 degree 3 poles (36.9035, -44.5374) (35.1678, -45.5188) (33.1775, -45.6076) (31.5191, -44.8193) (30.4628, -44.3172) (29.5504, -43.4745) (28.8905, -42.373) knots 0.019099 0.019099 0.019099 0.019099 0.618328 0.618328 0.618328 1 1 1 1
  spline S315 degree 3 poles (28.8905, -42.373) (28.2356, -41.2799) (28.0251, -39.987) (28.2891, -38.7134) (28.4327, -38.0204) (28.7011, -37.3303) (29.0737, -36.6286) knots 0 0 0 0 0.647645 0.647645 0.647645 1 1 1 1
  line L53 (29.0737, -36.6286) -> (29.1612, -36.4638)
  line L54 (29.1612, -36.4638) -> (28.9908, -36.2914)
  spline S316 degree 3 poles (28.9908, -36.2914) (28.3897, -35.6836) (27.931, -35.0843) (27.6841, -34.3672) (27.522, -33.8963) (27.4651, -33.4076) (27.4689, -32.9193) knots 0 0 0 0 0.603605 0.603605 0.603605 1 1 1 1
  spline S317 degree 3 poles (27.4689, -32.9193) (27.4781, -31.7149) (28.0681, -30.6219) (28.9533, -29.8689) (29.5522, -29.3594) (30.2878, -28.9905) (31.1058, -28.7908) knots 0 0 0 0 0.569109 0.569109 0.569109 0.954182 0.954182 0.954182 0.954182
  spline S318 degree 3 poles (31.1058, -28.7908) (31.1178, -28.4593) (31.1283, -28.0519) (31.1352, -27.6181) knots 0.607387 0.607387 0.607387 0.607387 1 1 1 1
  spline S319 degree 3 poles (31.1352, -27.6181) (31.1644, -25.7831) (31.0814, -24.7731) (30.8193, -23.7418) (30.754, -23.485) (30.6766, -23.2243) (30.5839, -22.9462) knots 0 0 0 0 0.800641 0.800641 0.800641 1 1 1 1
  spline S320 degree 3 poles (30.5839, -22.9462) (29.9756, -21.1214) (28.9014, -19.8352) (27.6291, -19.2047) knots 0 0 0 0 1 1 1 1
  spline S321 degree 3 poles (27.6291, -19.2047) (26.8945, -18.8407) (26.4461, -18.7298) (25.9454, -18.7349) (25.7421, -18.7369) (25.5228, -18.7611) (25.2651, -18.8137) knots 0 0 0 0 0.711303 0.711303 0.711303 1 1 1 1
  spline S322 degree 3 poles (25.2651, -18.8137) (23.7232, -19.1281) (22.4595, -20.0877) (21.5265, -21.709) (21.0344, -22.5641) (20.647, -23.6026) (20.4034, -24.8024) knots 0 0 0 0 0.654705 0.654705 0.654705 1 1 1 1
  spline S323 degree 3 poles (20.4034, -24.8024) (20.2739, -25.4408) (20.1421, -26.5799) (20.0696, -27.6039) (20.0342, -28.1041) (20.0114, -28.5828) (20.0045, -28.9687) knots 0 0 0 0 0.457255 0.457255 0.457255 0.680586 0.680586 0.680586 0.680586
  spline S324 degree 3 poles (20.0045, -28.9687) (20.1737, -28.9716) (20.3641, -28.9728) (20.5728, -28.9721) knots 0.788153 0.788153 0.788153 0.788153 1 1 1 1
  spline S325 degree 3 poles (20.5728, -28.9721) (21.4581, -28.9695) (21.9205, -28.9661) (22.3941, -29.0471) (22.71, -29.1012) (22.9935, -29.2034) (23.2325, -29.3044) knots 0 0 0 0 0.599835 0.599835 0.599835 1 1 1 1
  spline S326 degree 3 poles (23.2325, -29.3044) (24.2399, -29.7303) (25.0756, -30.3613) (25.5649, -31.2416) (25.8255, -31.7103) (25.9766, -32.236) (26.0196, -32.7724) knots 0.000002 0.000002 0.000002 0.000002 0.65253 0.65253 0.65253 1 1 1 1
  spline S327 degree 3 poles (26.0196, -32.7724) (26.0464, -33.1056) (26.0575, -33.4303) (25.9898, -33.7774) (25.9304, -34.0819) (25.8237, -34.343) (25.7057, -34.6008) knots 0 0 0 0 0.532706 0.532706 0.532706 1 1 1 1
  spline S328 degree 3 poles (25.7057, -34.6008) (25.5195, -35.0076) (25.2776, -35.3845) (25.0063, -35.7274) knots 0 0 0 0 0.845752 0.845752 0.845752 0.845752
  spline S329 degree 3 poles (25.0063, -35.7274) (25.2152, -36.1653) (25.3445, -36.6528) (25.3876, -37.161) (25.3966, -37.268) (25.4033, -37.3773) (25.4085, -37.4918) knots 0.077995 0.077995 0.077995 0.077995 0.83962 0.83962 0.83962 1 1 1 1
  spline S330 degree 3 poles (25.4085, -37.4918) (25.4258, -37.868) (25.439, -38.1756) (25.3733, -38.5347) (25.3129, -38.8652) (25.1915, -39.151) (25.0593, -39.4265) (25.0387, -39.4695) (25.0174, -39.513) (24.9954, -39.5579) knots 0 0 0 0 0.484601 0.484601 0.484601 0.930484 0.930484 0.930484 1 1 1 1
  spline S331 degree 3 poles (24.9954, -39.5579) (24.5918, -40.3776) (23.9772, -41.085) (23.1648, -41.5103) (22.385, -41.9186) (21.4967, -42.0784) (20.4603, -42.1269) knots 0 0 0 0 0.510228 0.510228 0.510228 1 1 1 1
  line L55 (20.4603, -42.1269) -> (20.1789, -42.1401)
  spline S332 degree 3 poles (20.1789, -42.1401) (19.8683, -42.9655) (19.3311, -43.6836) (18.669, -44.2614) (18.1917, -44.6778) (17.6457, -45.021) (17.0294, -45.2285) knots 0.1236 0.1236 0.1236 0.1236 0.632884 0.632884 0.632884 1 1 1 1
  spline S333 degree 3 poles (17.0294, -45.2285) (15.6679, -45.6868) (14.1945, -45.6326) (12.6935, -45.1125) (12.1298, -44.9172) (11.5566, -44.6602) (10.9624, -44.3448) knots 0 0 0 0 0.726997 0.726997 0.726997 1 1 1 1
  spline S334 degree 3 poles (10.9624, -44.3448) (10.8083, -44.263) (10.6793, -44.1929) (10.573, -44.1362) knots 0 0 0 0 0.122244 0.122244 0.122244 0.122244
  spline S335 degree 3 poles (10.573, -44.1362) (10.4946, -44.2052) (10.4022, -44.2872) (10.2936, -44.382) knots 0.893888 0.893888 0.893888 0.893888 1 1 1 1
  spline S336 degree 3 poles (10.2936, -44.382) (9.3884, -45.1716) (8.3652, -45.7598) (7.2449, -46.1286) knots 0 0 0 0 1 1 1 1
  spline S337 degree 3 poles (7.2449, -46.1286) (6.4114, -46.403) (5.4613, -46.5014) (4.5483, -46.4889) (3.8849, -46.4798) (3.2641, -46.4203) (2.6738, -46.2166) knots 0.000001 0.000001 0.000001 0.000001 0.579134 0.579134 0.579134 1 1 1 1